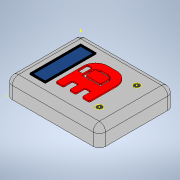
# Autodesk Inventor part: Part4
Saved by Autodesk Inventor 2020 (Build 240168000, 168)
## iProperties
Created: 2019-07-06
Part Number: Part4
Material: Generic
Document SubType Name: Sheet Metal
Designer: Gabriel Alves
Density: 1 g/cm^3
Sheet Metal Rule: Default
Appearance: Default
Author: Gabriel Alves
Autodesk Inventor part; units mm, degrees
ref_plane "YZ Plane" through (0, 0, 0) normal (1, 0, 0) x (0, 1, 0)
ref_plane "XZ Plane" through (0, 0, 0) normal (0, 1, 0) x (-1, 0, 0)
ref_plane "XY Plane" through (0, 0, 0) normal (0, 0, 1) x (1, 0, 0)
sketch "Sketch1" plane through (0, 0, 0) normal (0, 1, 0) x (-1, 0, 0)
  line L0 (0, 3048) -> (-3810, 3048)
  line L1 (-3810, 3048) -> (-3810, 0)
  line L2 (-3810, 0) -> (0, 0)
  line L3 (0, 0) -> (0, 3048)
  dimension "d0" = 3810
  dimension "d1" = 3048
  constraints: 8 end point, 2 parallel, 1 coincident, 1 horizontal, 1 perpendicular
  measures "d0" distance of L0.start L0.end
  measures "d1" distance of L0.end L1.end
extrude "Extrusion1" add sketch "Sketch1" along normal blind 762
sketch "Sketch2" plane through (0, 762, 0) normal (0, 1, 0) x (1, 0, 0)
  line L0 (482.6, -2565.4) -> (1117.6, -2565.4)
  line L1 (1117.6, -2565.4) -> (1117.6, -482.6)
  line L2 (1117.6, -482.6) -> (482.6, -482.6)
  line L3 (482.6, -482.6) -> (482.6, -2565.4)
  line L4 (0, -3048) -> (3810, -3048) projected
  line L5 (0, 0) -> (0, -3048) projected
  dimension "d5" = 2082.8
  dimension "d6" = 482.6
  dimension "d7" = 482.6
  dimension "d8" = 635
  constraints: 8 end point, 2 parallel, 1 horizontal, 1 perpendicular
  measures "d5" distance of L2.end L0.start
  measures "d6" distance between parallel lines of L4 L0
  measures "d7" distance between parallel lines of L5 L3
  measures "d8" distance of L1.end L2.end
extrude "Extrusion2" add sketch "Sketch2" along normal blind 50.8
sketch "Sketch3" plane through (0, 812.8, 0) normal (0, 1, 0) x (1, 0, 0)
  point P0 (0, 0)
sketch "Sketch4" plane through (0, 812.8, 0) normal (0, 1, 0) x (1, 0, 0)
  line L0 (533.4, -2514.6) -> (1066.8, -2514.6)
  line L1 (1066.8, -2514.6) -> (1066.8, -533.4)
  line L2 (1066.8, -533.4) -> (533.4, -533.4)
  line L3 (533.4, -533.4) -> (533.4, -2514.6)
  line L4 (482.6, -482.6) -> (482.6, -2565.4) projected
  line L5 (482.6, -2565.4) -> (1117.6, -2565.4) projected
  line L6 (1117.6, -2565.4) -> (1117.6, -482.6) projected
  line L7 (1117.6, -482.6) -> (482.6, -482.6) projected
  point P0 (0, 0)
  dimension "d11" = 50.8
  dimension "d12" = 50.8
  dimension "d13" = 50.8
  dimension "d14" = 50.8
  constraints: 8 end point, 2 parallel, 1 horizontal, 1 perpendicular
  measures "d11" distance between parallel lines of L5 L0
  measures "d12" distance between parallel lines of L7 L2
  measures "d13" distance between parallel lines of L6 L1
  measures "d14" distance between parallel lines of L4 L3
extrude "Extrusion3" cut sketch "Sketch4" against normal blind 50.8 contours L3 L2 L1 L0
fillet "Fillet1" radius 254 4 edges at (0, 381, 3048) (3810, 381, 3048) (3810, 381, 0) (0, 381, 0)
fillet "Fillet2" radius 254 8 edges at (0, 762, 1524) (74.3949, 762, 2973.6051) (1905, 762, 3048) (3735.6051, 762, 2973.6051) (3810, 762, 1524) (3735.6051, 762, 74.3949) (1905, 762, 0) (74.3949, 762, 74.3949)
sketch "Sketch5" plane through (0, 762, 0) normal (0, 1, 0) x (1, 0, 0)
  circle A0 centre (3048, -2286) radius 127
  circle A1 centre (3048, -762) radius 127
  line L0 (3556, -254) -> (3556, -2794) projected
  line L1 (254, -254) -> (3556, -254) projected
  line L2 (3556, -2794) -> (254, -2794) projected
  point P0 (0, 0)
  dimension "d19" = 254
  dimension "d20" = 508
  dimension "d21" = 508
  dimension "d22" = 508
  constraints: 2 centre point, 1 equal radius, 1 vertical alignment
  measures "d19" diameter of A0
  measures "d20" distance from line of L0 A0.centre
  measures "d21" distance from line of L1 A1.centre
  measures "d22" distance from line of L2 A0.centre
extrude "Extrusion4" cut sketch "Sketch5" against normal blind 254
sketch "Sketch6" plane through (3048, 508, 2286) normal (0, 1, 0) x (1, 0, 0)
  circle A0 centre (0, 0) radius 127 projected
  circle A1 centre (0, 1524) radius 127 projected
  line L0 (-124.4341, 25.4) -> (124.4341, 25.4)
  line L1 (-124.4341, -25.4) -> (124.4341, -25.4)
  line L2 (-25.4, -124.4341) -> (-25.4, 124.4341)
  line L3 (25.4, 124.4341) -> (25.4, -124.4341)
  circle A2 centre (0, 0) radius 127 projected
  line L4 (-124.4341, 1498.6) -> (124.4341, 1498.6)
  line L5 (124.4341, 1549.4) -> (-124.4341, 1549.4)
  line L6 (25.4, 1399.5659) -> (25.4, 1648.4341)
  line L7 (-25.4, 1399.5659) -> (-25.4, 1648.4341)
  point P0 (-3048, 2286)
  point P1 (-25.4, 1498.6)
  point P2 (25.4, 1498.6)
  point P3 (25.4, 1549.4)
  point P4 (-25.4, 1549.4)
  point P5 (25.4, -25.4)
  point P6 (25.4, 25.4)
  point P7 (-25.4, 25.4)
  point P8 (-25.4, -25.4)
  dimension "d25" = 50.8
  dimension "d26" = 50.8
  dimension "d27" = 25.4
  dimension "d28" = 25.4
  dimension "d29" = 25.4
  dimension "d30" = 25.4
  dimension "d31" = 50.8
  dimension "d32" = 50.8
  constraints: 16 end point, 3 parallel, 2 horizontal, 2 vertical, 1 perpendicular, 18 other
  measures "d25" distance between parallel lines of L0 L1
  measures "d26" distance between parallel lines of L3 L2
  measures "d27" distance from line of L1 point (0, 0)
  measures "d28" distance from line of L3 point (0, 0)
  measures "d29" distance from line of point (0, 1524) L7
  measures "d30" distance from line of L4 point (0, 1524)
  measures "d31" distance between parallel lines of L5 L4
  measures "d32" distance between parallel lines of L6 L7
extrude "Extrusion5" cut sketch "Sketch6" against normal blind 101.6 contours A0 L1 L3 L0 | L3 L0 L2 A0 | L3 L1 L2 L0 | A0 L2 L1 L3 | L2 L1 A0 L0 | A1 L4 L6 L5 | L6 L5 L7 A1 | L6 L4 L7 L5 | A1 L7 L4 L6 | L7 L4 A1 L5
sketch "Sketch7" plane through (0, 762, 0) normal (0, 1, 0) x (1, 0, 0)
  circle A0 centre (3048, -2286) radius 127 projected
  circle A1 centre (3048, -762) radius 127 projected
  point P0 (0, 0)
sketch "Sketch9" plane through (0, 762, 0) normal (0, 1, 0) x (1, 0, 0)
  line L0 (1320.8, -2336.8) -> (2692.4, -2336.8)
  line L1 (2692.4, -2336.8) -> (2692.4, -711.2)
  line L2 (2692.4, -711.2) -> (1320.8, -711.2)
  line L3 (1320.8, -711.2) -> (1320.8, -2336.8)
  line L4 (254, -3048) -> (3556, -3048) projected
  line L5 (1117.6, -2565.4) -> (1117.6, -482.6) projected
  line L6 (1625.6, -2336.8) -> (1625.6, -711.2)
  line L7 (2133.6, -2336.8) -> (2133.6, -711.2)
  line L8 (1879.6, -2336.8) -> (1879.6, -711.2)
  line L9 (2387.6, -2336.8) -> (2387.6, -711.2)
  line L10 (1625.6, -1955.8) -> (1879.6, -1955.8)
  line L11 (2133.6, -1955.8) -> (2387.6, -1955.8)
  line L12 (1625.6, -1016) -> (2387.6, -1016)
  line L13 (1625.6, -1574.8) -> (2387.6, -1574.8)
  line L14 (1701.8, -1498.6) -> (2311.4, -1498.6)
  line L15 (2311.4, -1498.6) -> (2311.4, -1092.2)
  line L16 (2311.4, -1092.2) -> (1701.8, -1092.2)
  line L17 (1701.8, -1092.2) -> (1701.8, -1498.6)
  line L18 (1371.6, -1498.6) -> (1574.8, -1498.6)
  line L19 (1574.8, -1498.6) -> (1574.8, -1092.2)
  line L20 (1574.8, -1092.2) -> (1371.6, -1092.2)
  line L21 (1371.6, -1092.2) -> (1371.6, -1498.6)
  point P0 (0, 0)
  point P1 (2260.6, -1955.8)
  dimension "d35" = 1625.6
  dimension "d36" = 1371.6
  dimension "d37" = 711.2
  dimension "d38" = 203.2
  dimension "d39" = 304.8
  dimension "d40" = 304.8
  dimension "d41" = 254
  dimension "d42" = 254
  dimension "d43" = 381
  dimension "d44" = 381
  dimension "d45" = 304.8
  dimension "d46" = 381
  dimension "d47" = 76.2
  dimension "d48" = 76.2
  dimension "d49" = 76.2
  dimension "d50" = 76.2
  dimension "d51" = 50.8
  dimension "d52" = 50.8
  constraints: 40 end point, 18 point on line, 9 perpendicular, 7 parallel, 4 horizontal, 1 midpoint
  measures "d35" distance between parallel lines of L2 L0
  measures "d36" distance between parallel lines of L1 L3
  measures "d37" distance between parallel lines of L4 L0
  measures "d38" distance between parallel lines of L5 L3
  measures "d39" distance between parallel lines of L3 L6
  measures "d40" distance between parallel lines of L1 L9
  measures "d41" distance between parallel lines of L9 L7
  measures "d42" distance between parallel lines of L7 L8
  measures "d43" distance between parallel lines of L10 L0
  measures "d44" distance between parallel lines of L0 L11
  measures "d45" distance between parallel lines of L2 L12
  measures "d46" distance between parallel lines of L13 L10
  measures "d47" distance between parallel lines of L6 L17
  measures "d48" distance between parallel lines of L9 L15
  measures "d49" distance between parallel lines of L13 L14
  measures "d50" distance between parallel lines of L12 L16
  measures "d51" distance between parallel lines of L6 L19
  measures "d52" distance between parallel lines of L3 L21
extrude "Extrusion6" add sketch "Sketch9" along normal blind 50.8 contours L3 L2 L6 L0 | L8 L13 L7 L0 | L6 L13 L8 L10 | L2 L8 L12 L6 | L2 L7 L12 L8 | L9 L2 L1 L0 | L7 L13 L9 L11 | L2 L9 L12 L7 | L14 L17 L16 L8 | L8 L16 L7 L14 | L7 L16 L15 L14
fillet "Fillet3" radius 508 2 edges at (2692.4, 787.4, 711.2) (1320.8, 787.4, 711.2)
fillet "Fillet4" radius 254 2 edges at (2387.6, 787.4, 1016) (1625.6, 787.4, 1016)
fillet "Fillet5" radius 50.8 18 edges at (1701.8, 787.4, 1092.2) (2311.4, 787.4, 1092.2) (2311.4, 787.4, 1498.6) (1701.8, 787.4, 1498.6) (1625.6, 787.4, 1955.8) (1879.6, 787.4, 1955.8) (1879.6, 787.4, 2336.8) (1320.8, 787.4, 2336.8) (1625.6, 787.4, 2336.8) (2133.6, 787.4, 2336.8) (2133.6, 787.4, 1955.8) (2387.6, 787.4, 1955.8) (2387.6, 787.4, 2336.8) (2692.4, 787.4, 2336.8) (1574.8, 787.4, 1092.2) (1371.6, 787.4, 1092.2) (1371.6, 787.4, 1498.6) (1574.8, 787.4, 1498.6)
sketch "Sketch10" plane through (254, 0, 3048) normal (0, 0, 1) x (1, 0, 0)
  point P0 (-254, 0)
equation "\"BendRadius\" = Thickness"
equation "\"BendReliefWidth\" = Thickness"
equation "\"BendReliefDepth\" = 0.5 * Thickness"
equation "\"CornerReliefSize\" = 4 * Thickness"
equation "\"MinimumRemnant\" = 2 * Thickness"
equation "\"TransitionRadius\" = BendRadius"
equation "\"JacobiRadiusSize\" = Thickness"
equation "\"GapSize\" = Thickness"
equation "\"Thickness\" = 3.048"
body "Solid1"
